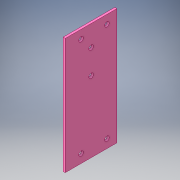
# Autodesk Inventor part: plate
Saved by Autodesk Inventor 2016 (Build 200138000, 138)
## iProperties
Created: 2016-03-02
Part Number: plate
Material: Generic
Document SubType Name: Modeling
Designer: gus
Density: 1 g/cm^3
Appearance: Pink
Author: gus
Autodesk Inventor part; units mm, degrees
ref_plane "YZ Plane" through (0, 0, 0) normal (1, 0, 0) x (0, 1, 0)
ref_plane "XZ Plane" through (0, 0, 0) normal (0, 1, 0) x (-1, 0, 0)
ref_plane "XY Plane" through (0, 0, 0) normal (0, 0, 1) x (1, 0, 0)
sketch "Sketch1" plane through (0, 0, 0) normal (1, 0, 0) x (0, 1, 0)
  line L0 (0, 0) -> (171.45, 0)
  line L1 (171.45, 0) -> (171.45, -76.2)
  line L2 (171.45, -76.2) -> (0, -76.2)
  line L3 (0, -76.2) -> (0, 0)
  dimension "d0" = 171.45
  dimension "d1" = 76.2
  constraints: 8 end point, 2 parallel, 1 horizontal, 1 perpendicular
  measures "d0" distance of L1.end L2.end
  measures "d1" distance of L2.end L0.start
extrude "Extrusion1" add sketch "Sketch1" along normal blind 3.175
sketch "Sketch2" plane through (0, 0, 0) normal (-1, 0, 0) x (0, 0, 1)
  circle A0 centre (-38.1, 140.6906) radius 3.3734
  line L0 (0, 171.45) -> (-76.2, 171.45) projected
  line L1 (0, 0) -> (0, 171.45) projected
  circle A1 centre (-38.1, 104.7696) radius 3.3734
  circle A2 centre (-61.4172, 12.7) radius 3.3734
  line L2 (-76.2, 171.45) -> (-76.2, 0) projected
  line L3 (0, 0) -> (-76.2, 0) projected
  circle A3 centre (-23.3172, 12.7) radius 3.3734
  circle A4 centre (-23.3172, 158.75) radius 3.3734
  circle A5 centre (-61.4172, 158.75) radius 3.3734
  dimension "d4" = 6.7469
  dimension "d5" = 30.7594
  dimension "d6" = 38.1
  dimension "d7" = 6.7469
  dimension "d8" = 38.1
  dimension "d9" = 35.921
  dimension "d12" = 6.7469
  dimension "d13" = 14.7828
  dimension "d14" = 12.7
  dimension "d15" = 6.7469
  dimension "d16" = 38.1
  dimension "d17" = 12.7
  dimension "d18" = 14.7828
  dimension "d19" = 38.1
  dimension "d20" = 12.7
  dimension "d21" = 12.7
  constraints: 6 centre point, 2 equal radius
  measures "d4" diameter of A0
  measures "d5" distance from line of L0 A0.centre
  measures "d6" distance from line of L1 A0.centre
  measures "d7" diameter of A1
  measures "d8" distance from line of L1 A1.centre
  measures "d9" distance of A0.centre A1.centre
  measures "d12" diameter of A2
  measures "d13" distance from line of L2 A2.centre
  measures "d14" distance from line of L3 A2.centre
  measures "d15" diameter of A3
  measures "d16" distance of A2.centre A3.centre
  measures "d17" distance from line of L3 A3.centre
  measures "d18" distance from line of L2 A5.centre
  measures "d19" distance of A4.centre A5.centre
  measures "d20" distance from line of L0 A5.centre
  measures "d21" distance from line of L0 A4.centre
extrude "Extrusion2" cut sketch "Sketch2" against normal blind 3.175 contours A0 | A1 | A2 | A3 | A4 | A5
body "Solid1"
